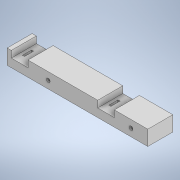
# Autodesk Inventor part: side_ToF_mount
Saved by Autodesk Inventor 2020 (Build 240168000, 168)
## iProperties
Created: 2022-07-20
Part Number: side_ToF_mount
Material: 일반
Document SubType Name: Modeling
Designer: SeungJin
Density: 1 g/cm^3
Appearance: 기본값
Author: SeungJin
Autodesk Inventor part; units mm, degrees
ref_plane "YZ Plane" through (0, 0, 0) normal (1, 0, 0) x (0, 1, 0)
ref_plane "XZ Plane" through (0, 0, 0) normal (0, 1, 0) x (-1, 0, 0)
ref_plane "작업 평면1" through (18, 12.5444, -60) normal (0, 0, -1) x (-1, 0, 0)
sketch "스케치1" plane through (18, 12.5444, -60) normal (0, 0, -1) x (-1, 0, 0)
  circle A0 centre (149.27, -9) radius 2.25 projected
  circle A1 centre (50, -9) radius 2.25 projected
  line L0 (60.4781, -35) -> (62.5565, -31.4) projected
  line L1 (62.5565, -31.4) -> (66.7134, -31.4) projected
  line L2 (66.7134, -31.4) -> (68.7919, -35) projected
  line L3 (68.7919, -35) -> (66.7134, -38.6) projected
  line L4 (66.7134, -38.6) -> (62.5565, -38.6) projected
  line L5 (62.5565, -38.6) -> (60.4781, -35) projected
  line L6 (161.8265, -38.6) -> (159.748, -35) projected
  line L7 (159.748, -35) -> (161.8265, -31.4) projected
  line L8 (161.8265, -31.4) -> (165.9834, -31.4) projected
  line L9 (165.9834, -31.4) -> (168.0619, -35) projected
  line L10 (168.0619, -35) -> (165.9834, -38.6) projected
  line L11 (165.9834, -38.6) -> (161.8265, -38.6) projected
  line L12 (30, -50) -> (198.5399, -50) projected
  line L13 (198.5399, -50) -> (198.5399, 0) projected
  line L14 (0, 0) -> (198.5399, 0) projected
  line L15 (0, 0) -> (0, -12.5444) projected
  line L16 (0, -12.5444) -> (30, -12.5444) projected
  line L17 (30, -12.5444) -> (30, -50) projected
  line L18 (30, 0) -> (30, -18)
  line L19 (30, -18) -> (198.5399, -18)
  line L20 (198.5399, -18) -> (198.5399, 0)
  line L21 (176.0399, 8) -> (191.0399, 8) projected
  line L22 (72.5, 8) -> (87.5, 8) projected
  line L23 (193.5399, -8) -> (173.5399, -8)
  line L24 (173.5399, -8) -> (173.5399, 0)
  line L25 (193.5399, 0) -> (193.5399, -8)
  line L26 (90, -8) -> (70, -8)
  line L27 (70, -8) -> (70, 0)
  line L28 (90, 0) -> (90, -8)
  line L29 (70, 0) -> (30, 0)
  line L30 (198.5399, 0) -> (193.5399, 0)
  line L31 (173.5399, 0) -> (90, 0)
  point P0 (18, -12.5444)
  point P1 (80, -8)
  point P2 (80, 8)
  point P3 (183.5399, -8)
  point P4 (183.5399, 8)
  point P5 (70, 0)
  dimension "d1" = 18
  dimension "d6" = 8
  dimension "d7" = 8
  constraints: 24 end point, 6 parallel, 5 horizontal, 5 perpendicular, 4 midpoint, 2 vertical alignment, 1 point on line
  measures "d1" distance of L18.end L18.start
  measures "d6" distance of L23.end L24.end
  measures "d7" distance of L28.start L26.start
extrude "돌출1" add sketch "스케치1" along normal blind 30 contours L17 L18 L14 L27 L26 L28 L24 L23 L25 L13 L19
sketch "스케치2" plane through (18, 12.5444, -90) normal (0, 0, -1) x (-1, 0, 0)
  circle A0 centre (149.27, -9) radius 2.25 projected
  circle A1 centre (50, -9) radius 2.25 projected
  circle A2 centre (149.27, -9) radius 4
  circle A3 centre (50, -9) radius 4
  point P0 (18, -12.5444)
  dimension "d10" = 8
  dimension "d11" = 8
  constraints: 2 centre point, 2 coincident
  measures "d10" diameter of A2
  measures "d11" diameter of A3
extrude "돌출2" cut sketch "스케치2" against normal blind 25 contours A0 | A1 | A2 | A3
sketch "스케치3" plane through (-175.5399, 4.5444, -60) normal (0, 1, 0) x (1, 0, 0)
  line L0 (0, 0) -> (20, 0) projected
  line L1 (20, 0) -> (20, 30) projected
  line L2 (0, 30) -> (20, 30) projected
  line L3 (0, 0) -> (0, 30) projected
  line L4 (103.5399, 0) -> (123.5399, 0) projected
  line L5 (123.5399, 0) -> (123.5399, 30) projected
  line L6 (103.5399, 30) -> (123.5399, 30) projected
  line L7 (103.5399, 0) -> (103.5399, 30) projected
  line L8 (5, 20.5) -> (15, 20.5)
  line L9 (15, 20.5) -> (15, 9.5)
  line L10 (15, 9.5) -> (5, 9.5)
  line L11 (5, 9.5) -> (5, 20.5)
  line L12 (5, 20.5) -> (15, 9.5) construction
  line L13 (15, 20.5) -> (5, 9.5) construction
  line L14 (108.5399, 20.5) -> (118.5399, 20.5)
  line L15 (118.5399, 20.5) -> (118.5399, 9.5)
  line L16 (118.5399, 9.5) -> (108.5399, 9.5)
  line L17 (108.5399, 9.5) -> (108.5399, 20.5)
  line L18 (108.5399, 20.5) -> (118.5399, 9.5) construction
  line L19 (118.5399, 20.5) -> (108.5399, 9.5) construction
  line L20 (3.75, 20.5) -> (6.25, 20.5)
  line L21 (6.25, 20.5) -> (6.25, 9.5)
  line L22 (6.25, 9.5) -> (3.75, 9.5)
  line L23 (3.75, 9.5) -> (3.75, 20.5)
  line L24 (3.75, 20.5) -> (6.25, 9.5) construction
  line L25 (6.25, 20.5) -> (3.75, 9.5) construction
  line L26 (13.75, 20.5) -> (16.25, 20.5)
  line L27 (16.25, 20.5) -> (16.25, 9.5)
  line L28 (16.25, 9.5) -> (13.75, 9.5)
  line L29 (13.75, 9.5) -> (13.75, 20.5)
  line L30 (13.75, 20.5) -> (16.25, 9.5) construction
  line L31 (16.25, 20.5) -> (13.75, 9.5) construction
  line L32 (107.2899, 20.5) -> (109.7899, 20.5)
  line L33 (109.7899, 20.5) -> (109.7899, 9.5)
  line L34 (109.7899, 9.5) -> (107.2899, 9.5)
  line L35 (107.2899, 9.5) -> (107.2899, 20.5)
  line L36 (107.2899, 20.5) -> (109.7899, 9.5) construction
  line L37 (109.7899, 20.5) -> (107.2899, 9.5) construction
  line L38 (117.2899, 20.5) -> (119.7899, 20.5)
  line L39 (119.7899, 20.5) -> (119.7899, 9.5)
  line L40 (119.7899, 9.5) -> (117.2899, 9.5)
  line L41 (117.2899, 9.5) -> (117.2899, 20.5)
  line L42 (117.2899, 20.5) -> (119.7899, 9.5) construction
  line L43 (119.7899, 20.5) -> (117.2899, 9.5) construction
  point P0 (175.5399, -60)
  point P1 (10, 15)
  point P2 (113.5399, 15)
  point P3 (5, 15)
  point P4 (15, 15)
  point P5 (108.5399, 15)
  point P6 (118.5399, 15)
  point P7 (118.5399, 20.5)
  point P8 (117.2899, 20.5)
  point P9 (117.2899, 9.5)
  point P10 (118.5399, 9.5)
  point P11 (108.5399, 9.5)
  point P12 (109.7899, 20.5)
  point P13 (108.5399, 20.5)
  point P14 (13.75, 20.5)
  point P15 (13.75, 9.5)
  point P16 (15, 9.5)
  point P17 (15, 20.5)
  point P18 (6.25, 20.5)
  point P19 (5, 20.5)
  point P20 (5, 9.5)
  dimension "d14" = 10
  dimension "d15" = 11
  dimension "d16" = 10
  dimension "d17" = 11
  dimension "d18" = 2.5
  dimension "d19" = 2.5
  dimension "d20" = 2.5
  dimension "d21" = 2.5
  constraints: 72 end point, 16 midpoint, 12 parallel, 6 horizontal, 6 perpendicular, 4 point on line
  measures "d14" distance of L9.end L10.end
  measures "d15" distance of L8.end L9.end
  measures "d16" distance of L15.end L16.end
  measures "d17" distance of L14.end L15.end
  measures "d18" distance of L21.end L22.end
  measures "d19" distance of L27.end L28.end
  measures "d20" distance of L33.end L34.end
  measures "d21" distance of L39.end L40.end
extrude "돌출3" cut sketch "스케치3" against normal through all contours L8 L21 L10 L11 | L11 L22 L23 L20 | L8 L9 L10 L29 | L26 L27 L28 L9 | L14 L33 L16 L17 | L17 L34 L35 L32 | L14 L15 L16 L41 | L38 L39 L40 L15
